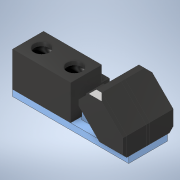
# Autodesk Inventor part: Sharp_Czujnik_Linia
Saved by Autodesk Inventor 2020 (Build 240168000, 168)
## iProperties
Created: 2019-01-30
Part Number: Sharp_Czujnik_Linia
Material: Ogólny
Document SubType Name: Modeling
Designer: atmat
Density: 1 g/cm^3
Appearance: Domyślna
Author: atmat
Autodesk Inventor part; units mm, degrees
ref_plane "YZ Plane" through (0, 0, 0) normal (1, 0, 0) x (0, 1, 0)
ref_plane "XZ Plane" through (0, 0, 0) normal (0, 1, 0) x (-1, 0, 0)
ref_plane "XY Plane" through (0, 0, 0) normal (0, 0, 1) x (1, 0, 0)
sketch "Szkic1" plane through (0, 0, 0) normal (0, 1, 0) x (-1, 0, 0)
  line L0 (7.5, 5) -> (-7.5, 5)
  line L1 (-7.5, 5) -> (-7.5, -5)
  line L2 (-7.5, -5) -> (7.5, -5)
  line L3 (7.5, -5) -> (7.5, 5)
  point P0 (0, 0)
  dimension "d0" = 10
  dimension "d1" = 15
  dimension "d2" = 5
  dimension "d3" = 7.5
  constraints: 8 end point, 2 parallel, 1 horizontal, 1 perpendicular
  measures "d0" distance of L2.end L0.start
  measures "d1" distance of L1.end L2.end
  measures "d2" distance from line of point (0, 0) L2
  measures "d3" distance from line of point (0, 0) L3
extrude "Wyciągnięcie proste1" add sketch "Szkic1" along normal blind 5
sketch "Szkic2" plane through (0, 5, 0) normal (0, 1, 0) x (1, 0, 0)
  line L0 (-7.5, -5) -> (7.5, -5) projected
  line L1 (7.5, -5) -> (7.5, 5) projected
  line L2 (-7.5, -5) -> (7.5, -5)
  line L3 (7.5, -5) -> (7.5, 3)
  line L4 (7.5, 3) -> (-7.5, 3)
  line L5 (-7.5, 3) -> (-7.5, -5)
  point P0 (0, 0)
  dimension "d6" = 8
  constraints: 8 end point, 2 parallel, 1 horizontal, 1 perpendicular, 1 point on line
  measures "d6" distance between parallel lines of L0 L4
extrude "Wyciągnięcie proste2" add sketch "Szkic2" along normal blind 4
sketch "Szkic3" plane through (0, 9, 0) normal (0, 1, 0) x (1, 0, 0)
  circle A0 centre (-4, -1) radius 2
  line L0 (-7.5, 3) -> (-7.5, -5) projected
  line L1 (7.5, 3) -> (-7.5, 3) projected
  circle A1 centre (4.5, -1) radius 2
  line L2 (7.5, -5) -> (7.5, 3) projected
  point P0 (0, 0)
  dimension "d9" = 4
  dimension "d10" = 3.5
  dimension "d11" = 4
  dimension "d12" = 3
  dimension "d13" = 4
  dimension "d14" = 4
  constraints: 2 centre point
  measures "d9" diameter of A0
  measures "d10" distance from line of L0 A0.centre
  measures "d11" distance from line of L1 A0.centre
  measures "d12" distance from line of L2 A1.centre
  measures "d13" distance from line of L1 A1.centre
  measures "d14" diameter of A1
extrude "Wyciągnięcie proste3" cut sketch "Szkic3" against normal blind 1
sketch "Sketch4" plane through (0, 0, 0) normal (0, -1, 0) x (1, 0, 0)
  line L0 (-7.5, 5) -> (7.5, 5) projected
  line L1 (7.5, -5) -> (-7.5, -5) projected
  line L2 (7.5, 5) -> (-7.5, 5)
  line L3 (-7.5, 5) -> (-7.5, -5)
  line L4 (-7.5, -5) -> (7.5, -5)
  line L5 (7.5, 5) -> (22.5, 5)
  line L6 (22.5, 5) -> (22.5, -5)
  line L7 (22.5, -5) -> (7.5, -5)
  line L8 (7.5, -5) -> (-7.5, -5) projected
  line L9 (-7.5, -5) -> (-7.5, 5) projected
  point P0 (0, 0)
  dimension "d19" = 30
  constraints: 12 end point, 4 equal length, 2 perpendicular, 1 horizontal
  measures "d19" distance between parallel lines of L3 L6
extrude "Extrusion4" add sketch "Sketch4" along normal blind 1.6 separate body
sketch "Sketch5" plane through (0, 0, 0) normal (0, 1, 0) x (1, 0, 0)
  line L0 (11.75, 2.85) -> (8.25, 2.85)
  line L1 (8.25, 2.85) -> (8.25, -2.85)
  line L2 (8.25, -2.85) -> (11.75, -2.85)
  line L3 (11.75, -2.85) -> (11.75, 2.85)
  line L4 (-7.5, 5) -> (22.5, 5) projected
  line L5 (7.5, -5) -> (7.5, 3) projected
  point P0 (0, 0)
  dimension "d20" = 3.5
  dimension "d21" = 5.7
  dimension "d22" = 2.15
  dimension "d23" = 0.75
  constraints: 8 end point, 2 parallel, 1 horizontal, 1 perpendicular
  measures "d20" distance of L1.end L2.end
  measures "d21" distance of L2.end L0.start
  measures "d22" distance between parallel lines of L4 L0
  measures "d23" distance between parallel lines of L5 L1
extrude "Extrusion5" add sketch "Sketch5" along normal blind 4.8 bodies 2
sketch "Sketch7" plane through (0, 4.8, 0) normal (0, 1, 0) x (1, 0, 0)
  line L0 (11.15, 2.2) -> (8.75, 2.2)
  line L1 (8.75, 2.2) -> (8.75, -2.2)
  line L2 (8.75, -2.2) -> (11.15, -2.2)
  line L3 (11.15, -2.2) -> (11.15, 2.2)
  line L4 (8.25, -2.85) -> (11.75, -2.85) projected
  line L5 (8.25, 2.85) -> (8.25, -2.85) projected
  point P0 (0, 0)
  dimension "d32" = 4.4
  dimension "d33" = 0.65
  dimension "d34" = 2.4
  dimension "d35" = 0.5
  constraints: 8 end point, 2 parallel, 1 horizontal, 1 perpendicular
  measures "d32" distance of L2.end L0.start
  measures "d33" distance between parallel lines of L4 L2
  measures "d34" distance of L1.end L2.end
  measures "d35" distance between parallel lines of L5 L1
extrude "Extrusion7" add sketch "Sketch7" along normal blind 1 bodies 2
ref_plane "Work Plane1" through (-7.5, 0, 3) normal (0, 0, 1) x (1, 0, 0)
ref_plane "Work Plane2" through (8.75, 4.8, 1.2) normal (0, 0, 1) x (1, 0, 0)
ref_plane "Work Plane3" through (11.15, 4.8, -1.2) normal (0, 0, -1) x (-1, 0, 0)
ref_plane "Work Plane4" through (-7.5, 0, 0) normal (0, 0, 1) x (1, 0, 0)
sketch "Sketch9" plane through (8.75, 4.8, 1.2) normal (0, 0, 1) x (1, 0, 0)
  line L0 (1.4, 1) -> (3.354852, 7.2)
  line L1 (3.354852, 7.2) -> (-0.954852, 7.2)
  line L2 (-0.954852, 7.2) -> (1, 1)
  line L3 (1, 1) -> (1.4, 1)
  line L4 (0, 1) -> (2.4, 1)
  line L5 (2.4, 0) -> (2.4, 1)
  line L6 (2.4, 1) -> (0, 1) construction
  line L7 (1.2, 1) -> (1.2, 8.086547) construction
  line L8 (-16.25, 4.2) -> (-1.25, 4.2) construction
  line L9 (1.2, 1) -> (1.2, 7.2)
  point P0 (-8.75, -4.8)
  dimension "d47" = 0.4
  dimension "d48" = 0
  dimension "d49" = 1
  dimension "d50" = 17.5
  dimension "d51" = 35
  dimension "d53" = 3
  constraints: 12 end point, 2 midpoint, 1 horizontal, 1 parallel, 1 vertical
  measures "d47" distance of L2.end L0.start
  measures "d48" distance between parallel lines of L4 L3
  measures "d49" distance from line of L5 L0.start
  measures "d50" angle of L0 L7
  measures "d51" angle of L0 L2
  measures "d53" distance between parallel lines of L8 L1
sketch "Sketch8" plane through (-7.5, 0, 3) normal (0, 0, 1) x (1, 0, 0)
  circle A0 centre (22.845637, 7.071068) radius 2.5
  line L0 (24.613404, 8.838835) -> (29.209598, 4.242641)
  line L1 (29.209598, 4.242641) -> (25.674064, 0.707107)
  line L2 (25.674064, 0.707107) -> (21.07787, 5.303301)
  line L3 (21.07787, 5.303301) -> (24.613404, 8.838835)
  line L4 (30, 0) -> (0, 0)
  line L5 (22.845637, 10.606602) -> (29.209598, 4.242641)
  line L6 (29.209598, 4.242641) -> (25.674064, 0.707107)
  line L7 (25.674064, 0.707107) -> (19.310103, 7.071068)
  line L8 (19.310103, 7.071068) -> (18.602996, 6.363961)
  line L9 (18.602996, 6.363961) -> (24.966957, 0)
  line L10 (24.966957, 0) -> (30, 0)
  line L11 (30, 0) -> (30, 4.866452)
  line L12 (30, 4.866452) -> (23.552743, 11.313708)
  line L13 (23.552743, 11.313708) -> (22.845637, 10.606602)
  line L14 (19.25, 0) -> (19.25, 4.8)
  line L15 (30, 0) -> (30, -1.6)
  line L16 (27.441831, 2.474874) -> (21.07787, 8.838835)
  point P0 (7.5, 0)
  point P1 (19.25, 0.8)
  dimension "d39" = 5
  dimension "d40" = 6.5
  dimension "d41" = 45
  dimension "d44" = 5
  dimension "d54" = 1
  dimension "d55" = 1
  dimension "d56" = 0
  dimension "d57" = 0
  dimension "d58" = 0
  dimension "d59" = 0
  dimension "d60" = 0
  dimension "d62" = 0
  dimension "d64" = 0.1178
  dimension "d65" = 0
  dimension "d66" = 0
  constraints: 28 end point, 9 perpendicular, 3 point on circle, 2 parallel, 1 centre point, 1 collinear, 1 midpoint
  measures "d39" diameter of A0
  measures "d40" distance of L0.start L0.end
  measures "d41" angle of L4 L2
  measures "d44" distance of L0.end L1.end
  measures "d54" distance of L12.end L5.start
  measures "d55" distance of L7.end L8.end
  measures "d56" distance between parallel lines of L2 L7
  measures "d57" distance between parallel lines of L5 L0
  measures "d58" distance edge to line of A0 L8
  measures "d59" distance edge to line of A0 L13
  measures "d60" distance between parallel lines of L1 L6
  measures "d62" distance between parallel lines of L4 L10
  measures "d64" distance from line of L1 L11.end
  measures "d65" distance from line of L9.end L1
  measures "d66" distance between parallel lines of L15 L11
revolve "Revolution1" add sketch "Sketch8" angle 360 about axis through (19.941831, 2.474874, 3) along (-0.7071068, 0.7071068, 0) separate body picked at (24.127784, 8.123299) picked at (21.813021, 8.365927) contours A0 L16 L3 | A0 L0 L1 L16 | L3 L16 A0
sketch "Sketch10" plane through (-7.5, 0, 3) normal (0, 0, 1) x (1, 0, 0)
  circle A0 centre (22.845637, 7.071068) radius 2.5
  line L0 (24.613404, 8.838835) -> (29.209598, 4.242641)
  line L1 (29.209598, 4.242641) -> (25.674064, 0.707107)
  line L2 (25.674064, 0.707107) -> (21.07787, 5.303301)
  line L3 (21.07787, 5.303301) -> (24.613404, 8.838835)
  line L4 (22.13853, 11.313708) -> (29.209598, 4.242641)
  line L5 (29.209598, 4.242641) -> (25.674064, 0.707107)
  line L6 (25.674064, 0.707107) -> (18.602996, 7.778175)
  line L7 (18.602996, 7.778175) -> (17.895889, 7.071068)
  line L8 (17.895889, 7.071068) -> (24.966957, 0)
  line L9 (24.966957, 0) -> (30, 0)
  line L10 (30, 0) -> (30, 4.866452)
  line L11 (30, 4.866452) -> (22.845637, 12.020815)
  line L12 (22.845637, 12.020815) -> (22.13853, 11.313708)
  line L13 (27.441831, 2.474874) -> (21.07787, 8.838835)
  point P0 (7.5, 0)
  dimension "d68" = 5
  dimension "d69" = 6.5
  dimension "d71" = 5
  dimension "d72" = 1
  dimension "d73" = 1
  dimension "d74" = 0
  dimension "d75" = 0
  dimension "d76" = 1
  dimension "d77" = 1
  dimension "d78" = 0
  dimension "d80" = 0.1178
  dimension "d81" = 0
  constraints: 28 end point, 9 perpendicular, 3 point on circle, 2 parallel, 1 centre point, 1 midpoint
  measures "d68" diameter of A0
  measures "d69" distance of L0.start L0.end
  measures "d71" distance of L0.end L1.end
  measures "d72" distance of L11.end L4.start
  measures "d73" distance of L6.end L7.end
  measures "d74" distance between parallel lines of L2 L6
  measures "d75" distance between parallel lines of L4 L0
  measures "d76" distance edge to line of A0 L7
  measures "d77" distance edge to line of A0 L12
  measures "d78" distance between parallel lines of L1 L5
  measures "d80" distance from line of L1 L10.end
  measures "d81" distance from line of L8.end L1
extrude "Extrusion8" add sketch "Sketch10" against normal mid plane 5 separate body contours L4 L12 L11 L10 L9 L8 L7 L6 L2 L1 L0
mirror "Mirror1" about plane through (-7.5, 0, 0) normal (0, 0, 1) of "Extrusion8", "Revolution1" bodies 4
chamfer "Chamfer1" distance 1 angle 45 4 edges at (15.3456, 12.0208, 3) (10.3959, 7.0711, 3) (10.3959, 7.0711, -3) (15.3456, 12.0208, -3)
sketch "Sketch12" plane through (-7.5, 0, 0) normal (0, 0, 1) x (1, 0, 0)
  line L0 (18.602996, 6.363961) -> (18.602996, 7.778175)
  line L1 (18.602996, 7.778175) -> (18.602996, 6.363961)
  line L2 (18.602996, 6.363961) -> (24.966957, 0)
  line L3 (0, 0) -> (30, 0)
  line L4 (24.966957, 0) -> (30, 0)
  line L5 (30, 0) -> (30, 4.866452)
  line L6 (23.552743, 11.313708) -> (30, 4.866452)
  line L7 (30, 4.866452) -> (23.552743, 11.313708)
  line L8 (29.209598, 4.242641) -> (22.13853, 11.313708)
  line L9 (23.552743, 11.313708) -> (22.13853, 11.313708)
  line L10 (22.13853, 11.313708) -> (18.602996, 7.778175)
  line L11 (18.602996, 6.363961) -> (24.966957, 0)
  line L12 (24.966957, 0) -> (30, 0)
  point P0 (7.5, 0)
  point P1 (24.966957, 0)
  constraints: 14 end point, 4 collinear, 2 perpendicular, 1 parallel
extrude "Extrusion11" add sketch "Sketch12" along normal mid plane 1 separate body
mirror "Mirror4" about plane through (-7.5, 0, 3) normal (0, 0, 1) of "Extrusion11" bodies 2
sketch "Sketch13" plane through (22.5, 0, -5.5) normal (0, 0, -1) x (-1, 0, 0)
  line L0 (11.397004, 7.778175) -> (11.397004, 6.363961)
  line L1 (11.397004, 7.778175) -> (11.397004, 6.363961)
  line L2 (5.033043, 0) -> (0, 0)
  line L3 (11.397004, 6.363961) -> (5.033043, 0)
  line L4 (5.033043, 0) -> (0, 0)
  line L5 (0, 4.866452) -> (6.447257, 11.313708)
  line L6 (0, 0) -> (0, 4.866452)
  line L7 (0, 4.866452) -> (6.447257, 11.313708)
  line L8 (6.447257, 11.313708) -> (7.86147, 11.313708)
  line L9 (7.86147, 11.313708) -> (11.397004, 7.778175)
  point P0 (22.5, 0)
  constraints: 14 end point, 3 collinear, 2 perpendicular, 1 parallel
extrude "Extrusion12" add sketch "Sketch13" along normal blind 1 bodies 4
chamfer "Chamfer2" distance 1 angle 45 2 edges at (19.9835, 0, 6.5) (19.9835, 0, -6.5)
chamfer "Chamfer3" distance 1 angle 45 2 edges at (15.3456, 11.3137, 6.5) (15.3456, 11.3137, -6.5)
body "Solid2"
body "Solid3"
body "Solid4"
body "Solid6"
